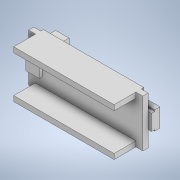
# Autodesk Inventor part: NANO
Saved by Autodesk Inventor 2022 (Build 260153070, 153G)
## iProperties
Created: 2021-11-30
Part Number: NANO
Material: Generic
Document SubType Name: Modeling
Designer: a laptop
Density: 1 g/cm^3
Appearance: Default
Author: a laptop
Autodesk Inventor part; units mm, degrees
ref_plane "YZ Plane" through (0, 0, 0) normal (1, 0, 0) x (0, 1, 0)
ref_plane "XZ Plane" through (0, 0, 0) normal (0, 1, 0) x (-1, 0, 0)
ref_plane "XY Plane" through (0, 0, 0) normal (0, 0, 1) x (1, 0, 0)
sketch "Sketch1" plane through (0, 0, 0) normal (0, 0, 1) x (1, 0, 0)
  line L0 (0, 18) -> (43.25, 18)
  line L1 (43.25, 18) -> (43.25, 0)
  line L2 (43.25, 0) -> (0, 0)
  line L3 (0, 0) -> (0, 9)
  line L4 (0, 12.81) -> (5.08, 12.81)
  line L5 (5.08, 12.81) -> (5.08, 5.19)
  line L6 (5.08, 5.19) -> (0, 5.19)
  line L7 (0, 5.19) -> (0, 9)
  line L8 (0, 9) -> (43.25, 9) construction
  line L9 (0, 9) -> (0, 18)
  line L10 (0, 9) -> (0, 12.81)
  dimension "d0" = 43.25
  dimension "d1" = 18
  dimension "d3" = 7.62
  dimension "d4" = 5.08
  constraints: 22 end point, 5 parallel, 3 horizontal, 2 collinear, 2 perpendicular, 2 point on line, 1 coincident, 1 midpoint, 1 vertical
  measures "d0" distance of L0.start L0.end
  measures "d1" distance of L0.end L1.end
  measures "d3" distance of L4.end L5.end
  measures "d4" distance of L4.start L4.end
extrude "Extrusion1" add sketch "Sketch1" along normal blind 2 contours L0 L1 L2 L3 L6 L5 L4 L9
extrude "Extrusion2" add sketch "Sketch1" along normal blind 3 and the other way blind 8.25 contours L4 L5 L6 L3 L9
sketch "Sketch2" plane through (43.25, 0, 0) normal (1, 0, 0) x (0, 0, -1)
  line L0 (0, 12) -> (1.25, 12)
  line L1 (1.25, 6) -> (0, 6)
  line L2 (0, 6) -> (0, 9)
  line L3 (3.25, 5.5) -> (1.25, 5.5)
  line L4 (1.25, 5.5) -> (1.25, 6)
  line L5 (1.25, 12.5) -> (3.25, 12.5)
  line L6 (3.25, 12.5) -> (3.25, 5.5)
  line L7 (0, 9) -> (3.25, 9) construction
  line L8 (0, 9) -> (0, 12)
  line L9 (1.25, 9) -> (1.25, 12) construction
  line L10 (1.25, 12) -> (1.25, 12.5)
  line L11 (1.25, 6) -> (1.25, 9) construction
  line L12 (0, 18) -> (0, 0) projected
  line L13 (0, 0) -> (0, 18) projected
  point P0 (0, 12.81)
  point P1 (0, 5.19)
  point P2 (0, 9)
  point P3 (0, 9)
  dimension "d9" = 6
  dimension "d10" = 1.25
  dimension "d12" = 7
  dimension "d13" = 2
  constraints: 24 end point, 7 perpendicular, 6 parallel, 2 collinear, 2 horizontal, 2 midpoint, 2 point on line, 1 coincident, 1 horizontal alignment, 2 other
  measures "d9" distance of L1.end L0.start
  measures "d10" distance of L0.start L0.end
  measures "d12" distance of L5.end L3.start
  measures "d13" distance of L5.start L5.end
extrude "Extrusion3" add sketch "Sketch2" along normal blind 1.25 and the other way blind 8
sketch "Sketch3" plane through (0, 0, 2) normal (0, 0, 1) x (1, 0, 0)
  line L0 (2.625, 18) -> (40.625, 18)
  line L1 (40.625, 18) -> (40.625, 16)
  line L2 (40.625, 16) -> (2.625, 16)
  line L3 (2.625, 16) -> (2.625, 18)
  line L4 (0, 18) -> (0, 12.81) projected
  line L5 (2.625, 17) -> (0, 18) construction
  line L6 (40.625, 17) -> (43.25, 18) construction
  line L7 (43.25, 0) -> (43.25, 18) projected
  line L8 (43.25, 9) -> (0, 9) construction
  line L9 (0, 5.19) -> (0, 12.81) projected
  line L10 (2.625, 0) -> (40.625, 0)
  line L11 (40.625, 0) -> (40.625, 2)
  line L12 (40.625, 2) -> (2.625, 2)
  line L13 (2.625, 2) -> (2.625, 0)
  point P0 (0, 0)
  dimension "d20" = 38
  dimension "d21" = 2
  constraints: 22 end point, 4 midpoint, 4 symmetric about line, 2 parallel, 1 coincident, 1 equal length, 1 horizontal, 1 horizontal alignment, 1 perpendicular
  measures "d20" distance of L0.start L0.end
  measures "d21" distance of L0.end L1.end
extrude "Extrusion4" add sketch "Sketch3" along normal blind 8.25 and the other way blind 3
body "Solid1"
